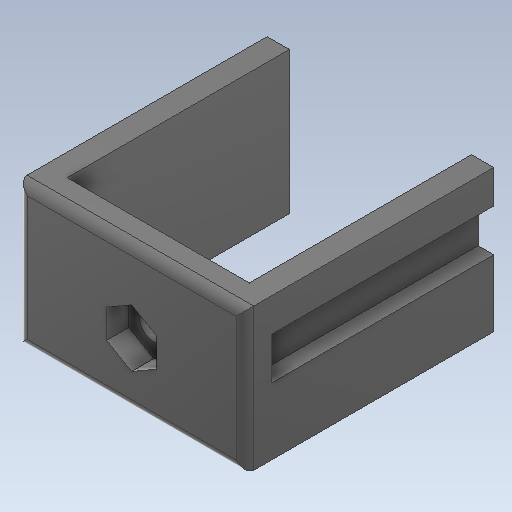
# Autodesk Inventor part: kicker_head_flat
Saved by Autodesk Inventor 2020 (Build 240168000, 168)
## iProperties
Created: 2023-12-16
Part Number: kicker_head_flat
Material: Типовые
Document SubType Name: Modeling
Designer: denis
Density: 1 g/cm^3
Appearance: Гладкая — черная
Author: denis
## iProperties of the stored document _3DПЕЧАТЬ.ipt
Created: 2024-02-02
Part Number: _3DПЕЧАТЬ
Material: Типовые
Document SubType Name: Modeling
Designer: 4s
Density: 1 g/cm^3
Appearance: По умолчанию
Author: 4s
Autodesk Inventor part; units mm, degrees
ref_plane "YZ Plane" through (0, 0, 0) normal (1, 0, 0) x (0, 1, 0)
ref_plane "XZ Plane" through (0, 0, 0) normal (0, 1, 0) x (-1, 0, 0)
ref_plane "XY Plane" through (0, 0, 0) normal (0, 0, 1) x (1, 0, 0)
sketch "Эскиз1" plane through (0, 0, 0) normal (0, 1, 0) x (-1, 0, 0)
  line L0 (0, 56.6418) -> (23.7825, 76.5969) construction
  line L1 (44.1942, 76.014) -> (76.014, 44.1942) construction
  line L2 (91.1, 52.2091) -> (52.2091, 91.1) construction
  line L3 (0, 0) -> (74.2462, 74.2462) construction
  arc A0 (92.5543, 49.5852) -> (48.7014, 93.0224) centre (0, 0) ccw construction
  line L4 (52.2091, 91.1) -> (48.6736, 87.5645) construction
  arc A1 (44.1942, 83.085) -> (44.1942, 76.014) centre (47.7297, 79.5495) ccw construction
  line L5 (52.2091, 91.1) -> (48.6736, 87.5645) construction
  line L6 (48.6736, 87.5645) -> (52.2091, 91.1) construction
  spline S0 degree 2 poles (48.6736, 87.5645) (52.2091, 91.1) (48.7014, 93.0224) knots 1 1 1 2 2 2 construction
  line L7 (52.2091, 91.1) -> (48.7014, 93.0224) construction
  line L8 (52.2091, 91.1) -> (48.7014, 93.0224) construction
  arc A2 (48.7014, 93.0224) -> (44.0271, 95.3237) centre (0, 0) ccw construction
  arc A3 (44.0271, 95.3237) -> (43.577, 95.5303) centre (0, 0) ccw construction
  line L9 (42.6652, 95.941) -> (43.577, 95.5303) construction
  line L10 (42.6652, 95.941) -> (43.577, 95.5303) construction
  spline S1 degree 2 poles (42.0492, 94.5734) (42.6652, 95.941) (43.577, 95.5303) knots 1 1 1 2 2 2 construction
  line L11 (42.0492, 94.5734) -> (42.6652, 95.941) construction
  line L12 (42.6652, 95.941) -> (42.0492, 94.5734) construction
  line L13 (0, 0) -> (0, 209.8821) construction
  spline S2 degree 2 poles (-48.6736, 87.5645) (-52.2091, 91.1) (-48.7014, 93.0224) knots 1 1 1 2 2 2 construction
  line L14 (-48.6736, 87.5645) -> (-52.2091, 91.1) construction
  line L15 (-52.2091, 91.1) -> (-48.7014, 93.0224) construction
  arc A4 (-44.1942, 76.014) -> (-44.1942, 83.085) centre (-47.7297, 79.5495) ccw construction
  line L16 (-44.1942, 76.014) -> (-76.014, 44.1942) construction
  arc A5 (-48.7014, 93.0224) -> (-92.5543, 49.5852) centre (0, 0) ccw construction
  arc A6 (-83.085, 44.1942) -> (-76.014, 44.1942) centre (-79.5495, 47.7297) ccw construction
  line L17 (-83.085, 44.1942) -> (-87.3563, 48.4654) construction
  spline S3 degree 2 poles (-48.6736, -87.5645) (-52.2091, -91.1) (-48.7014, -93.0224) knots 1 1 1 2 2 2 construction
  line L18 (-48.6736, -87.5645) -> (-52.2091, -91.1) construction
  line L19 (-52.2091, -91.1) -> (-48.7014, -93.0224) construction
  circle A7 centre (0, 0) radius 35 construction
  line L20 (-46.3155, -73.8927) -> (-73.8927, -46.3155) construction
  arc A8 (-73.8927, -46.3155) -> (-85.2064, -46.3155) centre (-79.5495, -51.9723) ccw construction
  line L21 (-85.2064, -46.3155) -> (-87.5645, -48.6736) construction
  line L22 (-87.5645, -48.6736) -> (-91.1, -52.2091) construction
  spline S4 degree 2 poles (-87.5645, -48.6736) (-91.1, -52.2091) (-92.5543, -49.5852) knots 1 1 1 2 2 2 construction
  line L23 (-91.1, -52.2091) -> (-92.5543, -49.5852) construction
  arc A9 (-92.5543, -49.5852) -> (-48.7014, -93.0224) centre (0, 0) ccw construction
  arc A10 (-92.5543, 49.5852) -> (-92.5543, -49.5852) centre (0, 0) ccw construction
  line L24 (48.6736, -87.5645) -> (46.3155, -85.2064) construction
  arc A11 (-46.3155, -85.2064) -> (-46.3155, -73.8927) centre (-51.9723, -79.5495) ccw construction
  line L25 (-48.6736, -87.5645) -> (-46.3155, -85.2064) construction
  arc A12 (-48.7014, -93.0224) -> (48.7014, -93.0224) centre (0, 0) ccw construction
  arc A13 (46.3155, -73.8927) -> (46.3155, -85.2064) centre (51.9723, -79.5495) ccw construction
  arc A14 (43.577, 95.5303) -> (-43.577, 95.5303) centre (0, 0) ccw construction
  arc A15 (23.7825, 76.5969) -> (0, 67.941) centre (0, 104.941) ccw construction
  line L26 (0, 56.6418) -> (-35.5516, 86.4744) construction
  line L27 (44.0271, 95.3237) -> (44.0271, 127.8162) construction
  ellipse E0 centre (0, 102.7511) end of major axis (44.0271, 102.7511) minor radius 27.5932 (42.0492, 94.5734) -> (35.2734, 86.2384) ccw construction
  line L28 (42.6652, 95.941) -> (-42.6652, 95.941) construction
  ellipse E1 centre (0, 102.7511) end of major axis (44.5159, 105.2445) minor radius 28.887 (35.2734, 86.2384) -> (42.0492, 94.5734) ccw construction
  line L29 (23.7825, 76.5969) -> (35.2734, 86.2384) construction
  arc A16 (0, 67.941) -> (23.7825, 76.5969) centre (0, 104.941) ccw construction
  arc A17 (-23.7825, 76.5969) -> (0, 67.941) centre (0, 104.941) ccw construction
  line L30 (-23.7825, 76.5969) -> (-35.2734, 86.2384) construction
  line L31 (-42.6652, 95.941) -> (-42.0492, 94.5734) construction
  arc A18 (-43.577, 95.5303) -> (-48.7014, 93.0224) centre (0, 0) ccw construction
  line L32 (-42.6652, 95.941) -> (-43.577, 95.5303) construction
  spline S5 degree 2 poles (-42.0492, 94.5734) (-42.6652, 95.941) (-43.577, 95.5303) knots 1 1 1 2 2 2 construction
  line L33 (-42.0492, 94.5734) -> (-42.6652, 95.941) construction
  line L34 (-42.6652, 95.941) -> (-43.577, 95.5303) construction
  line L35 (-42.6652, 95.941) -> (-43.577, 95.5303) construction
  spline S6 degree 2 poles (-42.0492, 94.5734) (-42.6652, 95.941) (-43.577, 95.5303) knots 1 1 1 2 2 2 construction
  line L36 (-42.0492, 94.5734) -> (-42.6652, 95.941) construction
  ellipse E2 centre (0, 102.7511) end of major axis (-44.5159, 105.2445) minor radius 28.887 (-42.0492, 94.5734) -> (-35.2734, 86.2384) ccw construction
  line L37 (83.085, 44.1942) -> (87.5645, 48.6736) construction
  arc A19 (76.014, 44.1942) -> (83.085, 44.1942) centre (79.5495, 47.7297) ccw construction
  spline S7 degree 2 poles (48.6736, -87.5645) (52.2091, -91.1) (48.7014, -93.0224) knots 1 1 1 2 2 2 construction
  line L38 (48.6736, -87.5645) -> (52.2091, -91.1) construction
  line L39 (52.2091, -91.1) -> (48.7014, -93.0224) construction
  line L40 (46.3155, -73.8927) -> (73.8927, -46.3155) construction
  arc A20 (85.2064, -46.3155) -> (73.8927, -46.3155) centre (79.5495, -51.9723) ccw construction
  line L41 (85.2064, -46.3155) -> (87.5645, -48.6736) construction
  spline S8 degree 2 poles (87.5645, -48.6736) (91.1, -52.2091) (92.5543, -49.5852) knots 1 1 1 2 2 2 construction
  line L42 (87.5645, -48.6736) -> (91.1, -52.2091) construction
  line L43 (91.1, -52.2091) -> (92.5543, -49.5852) construction
  arc A21 (92.5543, -49.5852) -> (92.5543, 49.5852) centre (0, 0) ccw construction
  arc A22 (48.7014, -93.0224) -> (92.5543, -49.5852) centre (0, 0) ccw construction
  arc A23 (28.5452, 71.4571) -> (-28.5452, 71.4571) centre (0, 104.941) ccw construction
  line L44 (-83.085, 34.2947) -> (-90.6891, 41.8987) construction
  line L45 (-93.5297, 47.6709) -> (-92.5543, 49.5852) construction
  line L46 (-29.1816, 81.127) -> (-76.014, 34.2947) construction
  arc A24 (-83.085, 34.2947) -> (-76.014, 34.2947) centre (-79.5495, 37.8302) ccw construction
  line L47 (-34.1491, 76.1596) -> (-28.5452, 71.4571) construction
  arc A25 (-30.6393, 73.2144) -> (-37.3889, 72.9198) centre (-33.8534, 69.3842) ccw construction
  arc A26 (-90.6891, 41.8987) -> (-87.3563, 48.4654) centre (0, 0) ccw construction
  arc A27 (37.3889, 72.9198) -> (30.6393, 73.2144) centre (33.8534, 69.3842) ccw construction
  line L48 (29.1816, 81.127) -> (76.014, 34.2947) construction
  arc A28 (76.014, 34.2947) -> (83.085, 34.2947) centre (79.5495, 37.8302) ccw construction
  line L49 (83.085, 34.2947) -> (90.6891, 41.8987) construction
  arc A29 (76.014, 44.1942) -> (83.085, 44.1942) centre (79.5495, 47.7297) ccw construction
  line L50 (44.1942, 76.014) -> (76.014, 44.1942) construction
  arc A30 (44.1942, 83.085) -> (44.1942, 76.014) centre (47.7297, 79.5495) ccw construction
  arc A31 (5.5413, 61.2914) -> (28.5452, 71.4571) centre (0, 104.941) ccw
  arc A32 (-28.5452, 71.4571) -> (5.5413, 61.2914) centre (0, 104.941) ccw
  line L51 (34.1491, 76.1596) -> (28.5452, 71.4571) construction
  arc A33 (-87.3563, 48.4654) -> (-90.6891, 41.8987) centre (0, 0) ccw construction
  line L52 (83.085, 44.1942) -> (87.3563, 48.4654) construction
  arc A34 (90.6891, 41.8987) -> (87.3563, 48.4654) centre (0, 0) ccw construction
  line L53 (-44.1942, 83.085) -> (-48.6736, 87.5645) construction
  line L54 (44.0271, 95.3237) -> (43.577, 95.5303) construction
  line L55 (48.6736, 87.5645) -> (44.1942, 83.085) construction
  line L56 (0, 104.941) -> (-23.6028, 54.3247) construction
  circle A35 centre (31.1916, 76.2887) radius 2 construction
  line L57 (29.1816, 81.127) -> (23.7825, 76.5969)
  line L58 (29.1816, 81.127) -> (34.1491, 76.1596)
  line L59 (34.1491, 76.1596) -> (28.5452, 71.4571)
  line L60 (-28.5452, 71.4571) -> (-34.1491, 76.1596)
  line L61 (-23.7825, 76.5969) -> (-29.1816, 81.127)
  line L62 (-29.1816, 81.127) -> (-34.1491, 76.1596)
  arc A36 (-26.6462, 78.9996) -> (-31.2232, 73.7044) centre (-28.9734, 76.3855) ccw
  arc A37 (31.2232, 73.7044) -> (26.6462, 78.9996) centre (28.9734, 76.3855) ccw
  line L63 (12.75, 58.0269) -> (-12.75, 58.0269)
  line L64 (0, 67.941) -> (0, 64.941) construction
  line L65 (-12.75, 58.0269) -> (-12.75, 67.2072) construction
  line L66 (12.75, 58.0269) -> (12.75, 67.2072) construction
  arc A38 (-12.75, 67.2072) -> (12.75, 67.2072) centre (0, 101.941) ccw
  line L67 (12.75, 67.2072) -> (12.75, 70.2072)
  line L68 (-12.75, 70.2072) -> (-12.75, 70.2072) construction
  line L69 (-12.75, 67.2072) -> (-12.75, 70.2072)
  line L70 (10.1, 59.4125) -> (-10.1, 59.4125) construction
  line L71 (12.75, 70.2072) -> (-12.75, 70.2072)
  line L72 (12.75, 67.2072) -> (-12.75, 67.2072)
  point P0 (60.1041, 60.1041)
  point P1 (40.6586, 79.5495)
  point P2 (79.5495, 40.6586)
  point P3 (0, 105)
  point P4 (-87.5645, 48.6736)
  point P5 (-23.542, 76.3968)
  point P6 (-34.9935, 86.0061)
  point P7 (0, 95.941)
  point P8 (-94.5192, 45.7288)
  point P9 (-13.2817, 58.6489)
  point P10 (-28.5452, 71.4571)
  point P11 (13.2817, 58.6489)
  point P12 (-15.6369, 71.4076)
  point P13 (-26.8032, 79.1314)
  point P14 (-31.2232, 73.7044)
  point P15 (26.8032, 79.1314)
  dimension "d67" = 44.5856
  dimension "d48" = 74
  dimension "d49" = 100
  dimension "d50" = 28
  dimension "d51" = 15
  dimension "d52" = 45
  dimension "d53" = 55
  dimension "d54" = 16.3348
  dimension "d55" = 27.5
  dimension "d56" = 5
  dimension "d57" = 5
  dimension "d58" = 1
  dimension "d59" = 1.5
  dimension "d60" = 1.5
  dimension "d61" = 1
  dimension "d62" = 4
  dimension "d63" = 70
  dimension "d64" = 85
  dimension "d65" = 105
  dimension "d66" = 1.3619
  dimension "d68" = 88
  dimension "d69" = 7
  dimension "d70" = 5
  dimension "d71" = 7
  dimension "d72" = 5
  dimension "d73" = 7
  dimension "d74" = 5
  dimension "d75" = 5.1
  dimension "d78" = 4
  dimension "d166" = 25.5
  dimension "d169" = 3
  dimension "d171" = 3
  dimension "d172" = 3
  dimension "d173" = 20.2
  constraints: 108 end point, 97 point on circle, 38 centre point, 30 horizontal alignment, 24 point on line, 21 coincident, 17 tangent, 11 collinear, 8 equal radius, 7 vertical, 5 parallel, 3 concentric, 3 horizontal, 3 perpendicular, 2 midpoint, 69 other
  measures "d48" diameter of A15
  measures "d49" angle of L26 L0
  measures "d50" distance from line of L28 L64.start
  measures "d51" distance of L0.end L29.end
  measures "d52" angle to the sketch x axis of L3
  measures "d53" distance of point (40.659, 79.55) point (79.55, 40.659)
  measures "d54" distance of L2.start point (79.55, 40.659)
  measures "d55" distance of point (40.659, 79.55) point (60.104, 60.104)
  measures "d56" radius of A1
  measures "d57" distance of L4.start L4.end
  measures "d58" distance of L12.start L10.end
  measures "d59" distance of L12.start L12.end
  measures "d60" distance of L31.start L31.end
  measures "d61" distance of L31.start L35.end
  measures "d62" distance of L4.start L7.end
  measures "d63" diameter of A7
  measures "d64" distance of point (60.104, 60.104) L3.start
  measures "d65" radius of A21
  measures "d66" distance from line of L27 L28.start
  measures "d68" diameter of A23
  measures "d69" distance between parallel lines of L17 L44
  measures "d70" radius of A6
  measures "d71" distance between parallel lines of L46 L16
  measures "d72" radius of A24
  measures "d73" distance between parallel lines of L26 L47
  measures "d74" radius of A25
  measures "d75" radial gap between concentric circles of A10 A26
  measures "d78" diameter of A35
  measures "d166" distance of L63.start L63.end
  measures "d169" distance of L64.start L64.end
  measures "d171" distance of L71.start L66.end
  measures "d172" distance of point (-12.75, 70.207) L65.end
  measures "d173" distance of L70.start L70.end
extrude "Выдавливание7" add sketch "Эскиз1" along normal blind 14 contours L69 L71 L67 L72
sketch "Эскиз10" plane through (12.75, 0, 67.2072) normal (0, 0, -1) x (-1, 0, 0)
  line L0 (25.5, 0) -> (0, 0) construction
  line L1 (0, 0) -> (0, 14) construction
  line L2 (25.5, 14) -> (0, 14) construction
  line L3 (25.5, 0) -> (25.5, 14) construction
  line L4 (25.5, 14) -> (0, 14) construction
  line L5 (12.75, 14) -> (12.75, 0) construction
  line L6 (-0.25, 15.8948) -> (-0.25, -2.2577) construction
  line L7 (0, 14) -> (2.5, 14)
  line L8 (2.5, 14) -> (2.5, 0)
  line L9 (2.5, 0) -> (0, 0)
  line L10 (0, 0) -> (0, 14)
  line L11 (0, 9) -> (2.5, 9) construction
  line L12 (0, 0) -> (0, 14) construction
  line L13 (0, 9.5) -> (1.75, 9.5)
  line L14 (1.75, 9.5) -> (1.75, 5.5)
  line L15 (1.75, 5.5) -> (0, 5.5)
  line L16 (0, 5.5) -> (0, 9.5) construction
  line L17 (0, 9) -> (1.25, 9) construction
  line L18 (1.25, 9) -> (1.25, 6) construction
  line L19 (1.25, 6) -> (0, 6) construction
  line L20 (0, 6) -> (0, 9) construction
  line L21 (1.25, 9) -> (0, 10.25)
  line L22 (25.5, 0) -> (25.5, 14) construction
  line L23 (25.5, 14) -> (23, 14)
  line L24 (23, 14) -> (23, 0)
  line L25 (23, 0) -> (25.5, 0)
  line L26 (25.5, 0) -> (25.5, 14)
  line L27 (25.5, 9) -> (23, 9) construction
  line L28 (25.5, 0) -> (25.5, 14) construction
  line L29 (25.5, 9.5) -> (23.75, 9.5)
  line L30 (23.75, 9.5) -> (23.75, 5.5)
  line L31 (23.75, 5.5) -> (25.5, 5.5)
  line L32 (25.5, 5.5) -> (25.5, 9.5) construction
  line L33 (25.5, 9) -> (24.25, 9) construction
  line L34 (24.25, 9) -> (24.25, 6) construction
  line L35 (24.25, 6) -> (25.5, 6) construction
  line L36 (25.5, 6) -> (25.5, 9) construction
  line L37 (24.25, 9) -> (25.5, 10.25)
  point P0 (24.75, 9.5)
  point P1 (0, 5.5)
  point P2 (0, 10.25)
  point P3 (0.75, 9.5)
  dimension "d215" = 26
  dimension "d216" = 20.5
  dimension "d218" = 3
  dimension "d219" = 1.5
  dimension "d220" = 0.5
  dimension "d221" = 0.5
  dimension "d222" = 0.5
  dimension "d223" = 135
  dimension "d237" = 5.5
  constraints: 64 end point, 14 symmetric about line, 9 point on line, 6 parallel, 5 perpendicular, 3 horizontal, 1 midpoint, 1 vertical
  measures "d215" diameter of L6 L5
  measures "d216" diameter of L8 L5
  measures "d218" distance of L17.end L18.end
  measures "d219" distance between parallel lines of L6 L18
  measures "d220" distance between parallel lines of L13 L17
  measures "d221" distance between parallel lines of L19 L15
  measures "d222" distance between parallel lines of L14 L18
  measures "d223" angle of L11 L21
  measures "d237" distance between parallel lines of L9 L15
extrude "Выдавливание16" add sketch "Эскиз10" along normal blind 25 contours L7 L8 L9 L10 L15 L14 L13 L21 | L26 L37 L29 L30 L31 L25 L24 L23
sketch "Эскиз12" plane through (-12.75, 0, 70.2072) normal (0, 0, 1) x (1, 0, 0)
  line L0 (0, 14) -> (2.5, 14) construction
  line L1 (2.5, 14) -> (2.5, 0) construction
  line L2 (2.5, 0) -> (0, 0) construction
  line L3 (0, 0) -> (0, 5.5) construction
  line L4 (0, 5.5) -> (1.75, 5.5) construction
  line L5 (1.75, 5.5) -> (1.75, 9.5) construction
  line L6 (1.75, 9.5) -> (0.75, 9.5) construction
  line L7 (0.75, 9.5) -> (0, 10.25) construction
  line L8 (0, 10.25) -> (0, 14) construction
  line L9 (0, 0) -> (25.5, 0) construction
  line L10 (25.5, 0) -> (25.5, 14) construction
  line L11 (0, 14) -> (25.5, 14) construction
  line L12 (0, 0) -> (0, 14) construction
  line L13 (25.5, 14) -> (25.5, 10.25) construction
  line L14 (25.5, 10.25) -> (24.75, 9.5) construction
  line L15 (24.75, 9.5) -> (23.75, 9.5) construction
  line L16 (23.75, 9.5) -> (23.75, 5.5) construction
  line L17 (23.75, 5.5) -> (25.5, 5.5) construction
  line L18 (25.5, 5.5) -> (25.5, 0) construction
  line L19 (25.5, 0) -> (23, 0) construction
  line L20 (23, 0) -> (23, 14) construction
  line L21 (23, 14) -> (25.5, 14) construction
  line L22 (23, 0) -> (23, 14) construction
  line L23 (0, 14) -> (25.5, 14) construction
  line L24 (23, 14) -> (25.5, 14) construction
  line L25 (23, 14) -> (2.5, 14) construction
  line L26 (0, 14) -> (2.5, 14) construction
  line L27 (25.5, 0) -> (25.5, 14) construction
  line L28 (25.5, 5.5) -> (25.5, 10.25) construction
  line L29 (0, 0) -> (0, 14) construction
  line L30 (0, 14) -> (25.5, 14) construction
  line L31 (12.75, 14) -> (12.75, 0) construction
  circle A0 centre (12.75, 5) radius 3.25
  circle A1 centre (12.75, 5) radius 1.65
  line L32 (12.75, 5) -> (15.5646, 6.625) construction
  line L33 (12.75, 5) -> (9.9354, 6.625) construction
  line L34 (12.75, 5) -> (16, 5) construction
  line L35 (12.75, 5) -> (15.5646, 3.375) construction
  line L36 (12.75, 5) -> (9.9354, 3.375) construction
  line L37 (15.5646, 6.625) -> (12.75, 8.25)
  line L38 (12.75, 8.25) -> (9.9354, 6.625)
  line L39 (9.9354, 6.625) -> (9.9354, 3.375)
  line L40 (15.5646, 6.625) -> (15.5646, 3.375)
  line L41 (15.5646, 3.375) -> (12.75, 1.75)
  line L42 (12.75, 1.75) -> (9.9354, 3.375)
  dimension "d226" = 6.5
  dimension "d229" = 3.3
  dimension "d238" = 5
  dimension "d239" = 60
  constraints: 24 end point, 4 symmetric about line, 3 point on circle, 3 vertical, 2 centre point, 2 point on line, 1 coincident, 1 horizontal, 2 other
  measures "d226" diameter of A0
  measures "d229" diameter of A1
  measures "d238" distance from line of L9 A0.centre
  measures "d239" angle of L31 L32
extrude "Выдавливание17" add sketch "Эскиз12" against normal blind 5.5 contours A0 L40 | L37 A0 | L40 L41 L42 L39 L38 L37 | A0 L41 | L38 A0 | A0 L42 | L39 A0 | A1
extrude "Выдавливание18" cut sketch "Эскиз12" against normal blind 5.5 contours A1
extrude "Выдавливание19" cut sketch "Эскиз12" against normal blind 2.5 contours L40 L41 L42 L39 L38 L37
fillet "Сопряжение1" [suppressed]
sketch "Эскиз14" plane through (0, 0, 0) normal (0, -1, 0) x (1, 0, 0)
  line L0 (-12.75, 70.2072) -> (12.75, 70.2072) projected
  line L1 (-12.75, 70.2072) -> (-12.75, 42.2072) projected
  line L2 (-10.25, 42.2072) -> (-12.75, 42.2072) projected
  line L3 (-10.25, 67.2072) -> (-10.25, 42.2072) projected
  line L4 (10.25, 67.2072) -> (-10.25, 67.2072) projected
  line L5 (10.25, 67.2072) -> (10.25, 42.2072) projected
  line L6 (12.75, 42.2072) -> (10.25, 42.2072) projected
  line L7 (12.75, 70.2072) -> (12.75, 42.2072) projected
  point P0 (0, 0)
extrude "Выдавливание20" add sketch "Эскиз14" along normal blind 2
fillet "Сопряжение2" radius 1 4 edges at (0, 14, 70.2072) (12.75, 6, 70.2072) (0, -2, 70.2072) (-12.75, 6, 70.2072)
